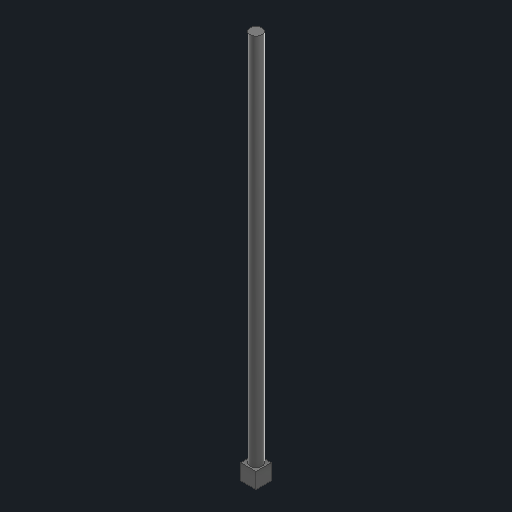
# Autodesk Inventor part: podstawa_rod
Saved by Autodesk Inventor 2027 (Build 310192060, 192F)
## iProperties
Created: 2026-08-24
Part Number: podstawa_rod
Material: Ogólny
Document SubType Name: Modeling
Designer: User
Density: 1 g/cm^3
Appearance: Domyślna
Author: User
Autodesk Inventor part; units mm, degrees
ref_plane "YZ Plane" through (0, 0, 0) normal (1, 0, 0) x (0, 1, 0)
ref_plane "XZ Plane" through (0, 0, 0) normal (0, 1, 0) x (-1, 0, 0)
ref_plane "XY Plane" through (0, 0, 0) normal (0, 0, 1) x (1, 0, 0)
sketch "Szkic1" plane through (0, 0, 0) normal (0, 1, 0) x (-1, 0, 0)
  line L0 (-4.9, 4.9) -> (4.9, 4.9)
  line L1 (4.9, 4.9) -> (4.9, -4.9)
  line L2 (4.9, -4.9) -> (-4.9, -4.9)
  line L3 (-4.9, -4.9) -> (-4.9, 4.9)
  line L4 (-4.9, 4.9) -> (4.9, -4.9) construction
  line L5 (4.9, 4.9) -> (-4.9, -4.9) construction
  circle A0 centre (0, 0) radius 3.9
  dimension "d0" = 9.8
  dimension "d1" = 9.8
  dimension "d2" = 7.8
  constraints: 12 end point, 2 midpoint, 2 parallel, 1 centre point, 1 coincident, 1 horizontal, 1 perpendicular
  measures "d0" distance of L1.end L2.end
  measures "d1" distance of L0.end L1.end
  measures "d2" diameter of A0
extrude "Wyciągnięcie proste1" add sketch "Szkic1" against normal blind 10 contours L0 L1 L2 L3 | A0
extrude "Wyciągnięcie proste2" add sketch "Szkic1" along normal blind 240 contours A0
